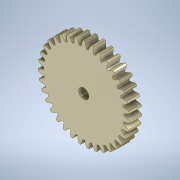
# Autodesk Inventor part: 正齒輪1
Saved by Autodesk Inventor 2020 (Build 240168000, 168)
## iProperties
CustomPartVersion: 1
Created: 2021-06-11
Part Number: 正齒輪1
Material: Steel
Document SubType Name: Modeling
Designer: user
Categories: <?xml version="1.0" encoding="UTF-16"?> <MemberInstance><Categories><FamilyTemplate><FamilyTemplateParameter ValueType="xs:double" Id="1" ObjectReferenceKey="da_z" ObjectType="kUserParameterObject"/><FamilyTemplateParameter ValueType="xs:double" Id="2" ObjectReferenceKey="da_b" ObjectType="kUserParameterObject"/><FamilyTemplateParameter ValueType="xs:double" Id="3" ObjectReferenceKey="da_beta" ObjectType="kUserParameterObject"/><FamilyTemplateParameter ValueType="xs:double" Id="4" ObjectReferenceKey="da_da" ObjectType="kUserParameterObject"/><FamilyTemplateParameter ValueType="xs:double" Id="5" ObjectReferenceKey="da_aw" ObjectType="kUserParameterObject"/><FamilyTemplateParameter ValueType="xs:string" Id="6" ObjectReferenceKey="EAIAABAAAACIAQAAAAAAAIAAAAAAAAAA" ObjectType="83910656" SubObjectId="SurfaceGeometry"/></FamilyTemplate><ParamToTemplateMap><ParamToTemplate CategoryParameter="//CategoryParameter[@InternalName='046C89C9-8512-4d59-83FE-43B91F4F132A']" TemplateParameter="1"/><ParamToTemplate CategoryParameter="//CategoryParameter[@InternalName='2552DF32-E462-4b46-AEBF-C6C7768E72AC']" TemplateParameter="2"/><ParamToTemplate CategoryParameter="//CategoryParameter[@InternalName='C9EE641D-15FC-4fae-A226-E94C4372FDD7']" TemplateParameter="3"/><ParamToTemplate><ParamToTemplate CategoryParameter="//CategoryParameter[@InternalName='00B6519A-459B-49c7-AD84-2E56D39A5744']" ConstantValue="0.000000"/></ParamToTemplate><ParamToTemplate><ParamToTemplate CategoryParameter="//CategoryParameter[@InternalName='04B31F0E-C7A6-4894-AA32-9629BEFACF47']" ConstantValue="1.000000"/></ParamToTemplate><ParamToTemplate><ParamToTemplate CategoryParameter="//CategoryParameter[@InternalName='43CBEC2E-7847-49e7-A936-2F7889FCB2D9']" ConstantValue="0.250000"/></ParamToTemplate><ParamToTemplate><ParamToTemplate CategoryParameter="//CategoryParameter[@InternalName='B1EFC894-105D-4ebd-86BF-FA20ED196853']" ConstantValue="0.350000"/></ParamToTemplate><ParamToTemplate><ParamToTemplate CategoryParameter="//CategoryParameter[@InternalName='51175063-3D10-4879-93E8-6246FE8B403D']" ConstantValue="2060000000.000000"/></ParamToTemplate><ParamToTemplate><ParamToTemplate CategoryParameter="//CategoryParameter[@InternalName='A3A52E27-4454-46a9-B0BD-C932399B70AF']" ConstantValue="0.300000"/></ParamToTemplate><ParamToTemplate><ParamToTemplate CategoryParameter="//CategoryParameter[@InternalName='91B76062-C214-41d9-B1B9-14D2AB99603D']" ConstantValue="0.200000"/></ParamToTemplate><ParamToTemplate><ParamToTemplate CategoryParameter="//CategoryParameter[@InternalName='374E806E-8B8A-4dda-A9AA-1039D6500AD2']" ConstantValue="5.000000"/></ParamToTemplate><ParamToTemplate><ParamToTemplate CategoryParameter="//CategoryParameter[@InternalName='2D373A89-B862-43d6-8D0B-0CBF12AB9F6C']" ConstantValue="0.349066"/></ParamToTemplate><ParamToTemplate CategoryParameter="//CategoryParameter[@InternalName='37777632-D6A2-4fac-9D53-DB8ACD95C989']" TemplateParameter="4"/><ParamToTemplate CategoryParameter="//CategoryParameter[@InternalName='FD1017F1-B727-4f7e-9707-0F86F1FF9423']" TemplateParameter="5"/><ParamToTemplate><ParamToTemplate CategoryParameter="//CategoryParameter[@InternalName='9E1B4470-B2D3-4ff1-B813-535BB4CDF51A']" ConstantValue="3520000.000000"/></ParamToTemplate><ParamToTemplate><ParamToTemplate CategoryParameter="//CategoryParameter[@InternalName='F8452263-BFF6-458c-9FB1-07C4B99E95CD']" ConstantValue="11400000.000000"/></ParamToTemplate><ParamToTemplate><ParamToTemplate CategoryParameter="//CategoryParameter[@InternalName='3E3BB259-FD49-497f-8171-6EBC954A3479']" ConstantValue="2.000000"/></ParamToTemplate><ParamToTemplate CategoryParameter="//CategoryParameter[@InternalName='27C3BAF2-7550-4e4b-AE2C-0DB134B7D9B7']" TemplateParameter="6"/></ParamToTemplateMap><Category DisplayName="Gear" InternalName="DC85795E-93AB-48d5-8EEE-5A27447B64BD" Mnemonic="Gear"><CategoryParameter DisplayName="z" InternalName="046C89C9-8512-4d59-83FE-43B91F4F132A" Mnemonic="z"/><CategoryParameter DisplayName="b" InternalName="2552DF32-E462-4b46-AEBF-C6C7768E72AC" Mnemonic="b"/><CategoryParameter DisplayName="||b|" InternalName="C9EE641D-15FC-4fae-A226-E94C4372FDD7" Mnemonic="beta"/><CategoryParameter DisplayName="x" InternalName="00B6519A-459B-49c7-AD84-2E56D39A5744" Mnemonic="x"/><CategoryParameter DisplayName="a*" InternalName="04B31F0E-C7A6-4894-AA32-9629BEFACF47" Mnemonic="a"/><CategoryParameter DisplayName="c*" InternalName="43CBEC2E-7847-49e7-A936-2F7889FCB2D9" Mnemonic="c"/><CategoryParameter DisplayName="r|.f|*" InternalName="B1EFC894-105D-4ebd-86BF-FA20ED196853" Mnemonic="rf"/><CategoryParameter DisplayName="E" InternalName="51175063-3D10-4879-93E8-6246FE8B403D" Mnemonic="E"/><CategoryParameter DisplayName="||m|" InternalName="A3A52E27-4454-46a9-B0BD-C932399B70AF" Mnemonic="mi"/><Category DisplayName="SpurGear" InternalName="26C5A22E-A91E-4dfd-A3B3-23CCAFAE1764" Mnemonic="SpurGear"><CategoryParameter DisplayName="m" InternalName="91B76062-C214-41d9-B1B9-14D2AB99603D" Mnemonic="m"/><CategoryParameter DisplayName="P" InternalName="374E806E-8B8A-4dda-A9AA-1039D6500AD2" Mnemonic="PP"/><CategoryParameter DisplayName="||a|" InternalName="2D373A89-B862-43d6-8D0B-0CBF12AB9F6C" Mnemonic="alpha"/><CategoryParameter DisplayName="d|.a|" InternalName="37777632-D6A2-4fac-9D53-DB8ACD95C989" Mnemonic="da"/><CategoryParameter DisplayName="a|.w|" InternalName="FD1017F1-B727-4f7e-9707-0F86F1FF9423" Mnemonic="aw"/><CategoryParameter DisplayName="||s||.Flim|" InternalName="9E1B4470-B2D3-4ff1-B813-535BB4CDF51A" Mnemonic="sFlim"/><CategoryParameter DisplayName="||s||.Hlim|" InternalName="F8452263-BFF6-458c-9FB1-07C4B99E95CD" Mnemonic="sHlim"/><CategoryParameter DisplayName="類型" InternalName="3E3BB259-FD49-497f-8171-6EBC954A3479" Mnemonic="type"/><CategoryParameter DisplayName="PitchDiameter" InternalName="27C3BAF2-7550-4e4b-AE2C-0DB134B7D9B7" Mnemonic="IDS_PITCHDIAM"/></Category></Category></Categories></MemberInstance>
Density: 1 g/cm^3
Appearance: 鎳
Author: user
Autodesk Inventor part; units mm, degrees
sketch "Sketch1" plane through (0, 0, 0) normal (0, 0, 1) x (1, 0, 0)
  circle A0 centre (0, 0) radius 37
  dimension "d0" = 74
  constraints: 1 centre point
  measures "d0" diameter of A0
extrude "Extrusion1" add sketch "Sketch1" along normal blind 20
ref_plane "Work Plane2" through (0, 0, 10) normal (0, 0, 1) x (1, 0, 0)
sketch "Sketch2" plane through (0, 0, 0) normal (0, 0, -1) x (-1, 0, 0)
  circle A0 centre (0, 0) radius 37 projected
  circle A1 centre (0, 0) radius 35
  dimension "d3" = 70
  constraints: 1 centre point, 1 coincident
  measures "d3" diameter of A1
surface extrude "節圓直徑" sketch "Sketch2" against normal through all shown no curves A1
ref_plane "Work Plane8" through (0, 0, 0) normal (0.9959743, 0.0896393, 0) x (0, 0, 1)
ref_plane "Work Plane9" through (0, 0, 0) normal (1, 0, 0) x (0, 1, 0)
spur gear teeth "正齒輪" teeth 35 pitch diameter 70 tip diameter 74 root diameter 65 face width 20 start plane through (0, 0, 0) normal (0, 0, -1) x (-1, 0, 0)
sketch "草圖3" plane through (0, 0, 20) normal (0, 0, 1) x (1, 0, 0)
  line L0 (-1.995, -3.467) -> (1.688, -3.6264) projected
  arc A0 (1.688, -3.6264) -> (-1.995, -3.467) centre (0, 0) ccw projected
  point P0 (0, 0)
ref_plane "工作平面11" through (-40.6499, -40.6499, -1.2) normal (0, 0, -1) x (0.0432397, 0.9990647, 0)
extrude "擠出2" cut sketch "草圖3" against normal up to surface (21.2 mm away)
sketch "草圖4" plane through (0, 0, 20) normal (0, 0, 1) x (1, 0, 0)
  line L0 (1.688, -3.6264) -> (-1.995, -3.467) projected
  arc A0 (1.688, -3.6264) -> (-1.995, -3.467) centre (0, 0) ccw projected
  arc A1 (-7.4218, 36.248) -> (-7.9411, 31.5149) centre (13.3274, 31.5766) ccw projected
  arc A2 (-7.9411, 31.5149) -> (-9.347, 31.1269) centre (0, 0) ccw projected
  arc A3 (-9.347, 31.1269) -> (-12.2203, 34.9237) centre (-27.6365, 20.2713) ccw projected
  arc A4 (-12.2203, 34.9237) -> (-13.7749, 34.3403) centre (0, 0) ccw projected
  arc A5 (-13.7749, 34.3403) -> (-13.4407, 29.5905) centre (7.475, 33.4489) ccw projected
  arc A6 (-13.4407, 29.5905) -> (-14.7547, 28.9577) centre (0, 0) ccw projected
  arc A7 (-14.7547, 28.9577) -> (-18.2598, 32.1804) centre (-30.812, 15.0108) ccw projected
  arc A8 (-18.2598, 32.1804) -> (-19.6852, 31.3288) centre (0, 0) ccw projected
  arc A9 (-19.6852, 31.3288) -> (-18.5082, 26.7151) centre (1.3824, 34.2461) ccw projected
  arc A10 (-18.5082, 26.7151) -> (-19.6882, 25.8578) centre (0, 0) ccw projected
  arc A11 (-19.6882, 25.8578) -> (-23.7124, 28.4029) centre (-32.9971, 9.2679) ccw projected
  arc A12 (-23.7124, 28.4029) -> (-24.9628, 27.3104) centre (0, 0) ccw projected
  arc A13 (-24.9628, 27.3104) -> (-22.981, 22.981) centre (-4.7547, 33.9425) ccw projected
  arc A14 (-22.981, 22.981) -> (-23.9889, 21.9268) centre (0, 0) ccw projected
  arc A15 (-23.9889, 21.9268) -> (-28.4029, 23.7124) centre (-34.1217, 3.2271) ccw projected
  arc A16 (-28.4029, 23.7124) -> (-29.4381, 22.4142) centre (0, 0) ccw projected
  arc A17 (-29.4381, 22.4142) -> (-26.7151, 18.5082) centre (-10.739, 32.5481) ccw projected
  arc A18 (-26.7151, 18.5082) -> (-27.5185, 17.291) centre (0, 0) ccw projected
  arc A19 (-27.5185, 17.291) -> (-32.1804, 18.2598) centre (-34.1496, -2.9174) ccw projected
  arc A20 (-32.1804, 18.2598) -> (-32.9672, 16.7976) centre (0, 0) ccw projected
  arc A21 (-32.9672, 16.7976) -> (-29.5905, 13.4407) centre (-16.3781, 30.1075) ccw projected
  arc A22 (-29.5905, 13.4407) -> (-30.1637, 12.0995) centre (0, 0) ccw projected
  arc A23 (-30.1637, 12.0995) -> (-34.9237, 12.2203) centre (-33.0798, -8.9682) ccw projected
  arc A24 (-34.9237, 12.2203) -> (-35.4368, 10.6412) centre (0, 0) ccw projected
  arc A25 (-35.4368, 10.6412) -> (-31.5149, 7.9411) centre (-21.4908, 26.6992) ccw projected
  arc A26 (-31.5149, 7.9411) -> (-31.8395, 6.5192) centre (0, 0) ccw projected
  arc A27 (-31.8395, 6.5192) -> (-36.5445, 5.7881) centre (-30.9469, -14.7307) ccw projected
  arc A28 (-36.5445, 5.7881) -> (-36.7674, 4.1427) centre (0, 0) ccw projected
  arc A29 (-36.7674, 4.1427) -> (-32.4264, 2.1862) centre (-25.9127, 22.4329) ccw projected
  arc A30 (-32.4264, 2.1862) -> (-32.4918, 0.7292) centre (0, 0) ccw projected
  arc A31 (-32.4918, 0.7292) -> (-36.9907, -0.8302) centre (-27.8193, -20.0197) ccw projected
  arc A32 (-36.9907, -0.8302) -> (-36.9162, -2.489) centre (0, 0) ccw projected
  arc A33 (-36.9162, -2.489) -> (-32.2956, -3.6388) centre (-29.5019, 17.4454) ccw projected
  arc A34 (-32.2956, -3.6388) -> (-32.0999, -5.0841) centre (0, 0) ccw projected
  arc A35 (-32.0999, -5.0841) -> (-36.248, -7.4218) centre (-23.7976, -24.6653) ccw projected
  arc A36 (-36.248, -7.4218) -> (-35.8785, -9.0406) centre (0, 0) ccw projected
  arc A37 (-35.8785, -9.0406) -> (-31.1269, -9.347) centre (-32.1428, 11.8973) ccw projected
  arc A38 (-31.1269, -9.347) -> (-30.6762, -10.7341) centre (0, 0) ccw projected
  arc A39 (-30.6762, -10.7341) -> (-34.3403, -13.7749) centre (-19.011, -28.5182) ccw projected
  arc A40 (-34.3403, -13.7749) -> (-33.6877, -15.3017) centre (0, 0) ccw projected
  arc A41 (-33.6877, -15.3017) -> (-28.9577, -14.7547) centre (-33.7506, 5.9668) ccw projected
  arc A42 (-28.9577, -14.7547) -> (-28.2666, -16.039) centre (0, 0) ccw projected
  arc A43 (-28.2666, -16.039) -> (-31.3288, -19.6852) centre (-13.6133, -31.4544) ccw projected
  arc A44 (-31.3288, -19.6852) -> (-30.4141, -21.0709) centre (0, 0) ccw projected
  arc A45 (-30.4141, -21.0709) -> (-25.8578, -19.6882) centre (-34.2736, -0.1555) ccw projected
  arc A46 (-25.8578, -19.6882) -> (-24.9485, -20.8285) centre (0, 0) ccw projected
  arc A47 (-24.9485, -20.8285) -> (-27.3104, -24.9628) centre (-7.7782, -33.3797) ccw projected
  arc A48 (-27.3104, -24.9628) -> (-26.163, -26.163) centre (0, 0) ccw projected
  arc A49 (-26.163, -26.163) -> (-21.9268, -23.9889) centre (-33.695, -6.2727) ccw projected
  arc A50 (-21.9268, -23.9889) -> (-20.8285, -24.9485) centre (0, 0) ccw projected
  arc A51 (-20.8285, -24.9485) -> (-22.4142, -29.4381) centre (-1.693, -34.2321) ccw projected
  arc A52 (-22.4142, -29.4381) -> (-21.0709, -30.4141) centre (0, 0) ccw projected
  arc A53 (-21.0709, -30.4141) -> (-17.291, -27.5185) centre (-32.0335, -12.1884) ccw projected
  arc A54 (-17.291, -27.5185) -> (-16.039, -28.2666) centre (0, 0) ccw projected
  arc A55 (-16.039, -28.2666) -> (-16.7976, -32.9672) centre (4.4466, -33.9843) ccw projected
  arc A56 (-16.7976, -32.9672) -> (-15.3017, -33.6877) centre (0, 0) ccw projected
  arc A57 (-15.3017, -33.6877) -> (-12.0995, -30.1637) centre (-29.3424, -17.7124) ccw projected
  arc A58 (-12.0995, -30.1637) -> (-10.7341, -30.6762) centre (0, 0) ccw projected
  arc A59 (-10.7341, -30.6762) -> (-10.6412, -35.4368) centre (10.4433, -32.6442) ccw projected
  arc A60 (-10.6412, -35.4368) -> (-9.0406, -35.8785) centre (0, 0) ccw projected
  arc A61 (-9.0406, -35.8785) -> (-6.5192, -31.8395) centre (-25.7082, -22.667) ccw projected
  arc A62 (-6.5192, -31.8395) -> (-5.0841, -32.0999) centre (0, 0) ccw projected
  arc A63 (-5.0841, -32.0999) -> (-4.1427, -36.7674) centre (16.1043, -30.2548) ccw projected
  arc A64 (-4.1427, -36.7674) -> (-2.489, -36.9162) centre (0, 0) ccw projected
  arc A65 (-2.489, -36.9162) -> (-0.7292, -32.4918) centre (-21.2477, -26.8931) ccw projected
  arc A66 (-0.7292, -32.4918) -> (0.7292, -32.4918) centre (0, 0) ccw projected
  arc A67 (0.7292, -32.4918) -> (2.489, -36.9162) centre (21.2477, -26.8931) ccw projected
  arc A68 (2.489, -36.9162) -> (4.1427, -36.7674) centre (0, 0) ccw projected
  arc A69 (4.1427, -36.7674) -> (5.0841, -32.0999) centre (-16.1043, -30.2548) ccw projected
  arc A70 (5.0841, -32.0999) -> (6.5192, -31.8395) centre (0, 0) ccw projected
  arc A71 (6.5192, -31.8395) -> (9.0406, -35.8785) centre (25.7082, -22.667) ccw projected
  arc A72 (9.0406, -35.8785) -> (10.6412, -35.4368) centre (0, 0) ccw projected
  arc A73 (10.6412, -35.4368) -> (10.7341, -30.6762) centre (-10.4433, -32.6442) ccw projected
  arc A74 (10.7341, -30.6762) -> (12.0995, -30.1637) centre (0, 0) ccw projected
  arc A75 (12.0995, -30.1637) -> (15.3017, -33.6877) centre (29.3424, -17.7124) ccw projected
  arc A76 (15.3017, -33.6877) -> (16.7976, -32.9672) centre (0, 0) ccw projected
  arc A77 (16.7976, -32.9672) -> (16.039, -28.2666) centre (-4.4466, -33.9843) ccw projected
  arc A78 (16.039, -28.2666) -> (17.291, -27.5185) centre (0, 0) ccw projected
  arc A79 (17.291, -27.5185) -> (21.0709, -30.4141) centre (32.0335, -12.1884) ccw projected
  arc A80 (21.0709, -30.4141) -> (22.4142, -29.4381) centre (0, 0) ccw projected
  arc A81 (22.4142, -29.4381) -> (20.8285, -24.9485) centre (1.693, -34.2321) ccw projected
  arc A82 (20.8285, -24.9485) -> (21.9268, -23.9889) centre (0, 0) ccw projected
  arc A83 (21.9268, -23.9889) -> (26.163, -26.163) centre (33.695, -6.2727) ccw projected
  arc A84 (26.163, -26.163) -> (27.3104, -24.9628) centre (0, 0) ccw projected
  arc A85 (27.3104, -24.9628) -> (24.9485, -20.8285) centre (7.7782, -33.3797) ccw projected
  arc A86 (24.9485, -20.8285) -> (25.8578, -19.6882) centre (0, 0) ccw projected
  arc A87 (25.8578, -19.6882) -> (30.4141, -21.0709) centre (34.2736, -0.1555) ccw projected
  arc A88 (30.4141, -21.0709) -> (31.3288, -19.6852) centre (0, 0) ccw projected
  arc A89 (31.3288, -19.6852) -> (28.2666, -16.039) centre (13.6133, -31.4544) ccw projected
  arc A90 (28.2666, -16.039) -> (28.9577, -14.7547) centre (0, 0) ccw projected
  arc A91 (28.9577, -14.7547) -> (33.6877, -15.3017) centre (33.7506, 5.9668) ccw projected
  arc A92 (33.6877, -15.3017) -> (34.3403, -13.7749) centre (0, 0) ccw projected
  arc A93 (34.3403, -13.7749) -> (30.6762, -10.7341) centre (19.011, -28.5182) ccw projected
  arc A94 (30.6762, -10.7341) -> (31.1269, -9.347) centre (0, 0) ccw projected
  arc A95 (31.1269, -9.347) -> (35.8785, -9.0406) centre (32.1428, 11.8973) ccw projected
  arc A96 (35.8785, -9.0406) -> (36.248, -7.4218) centre (0, 0) ccw projected
  arc A97 (36.248, -7.4218) -> (32.0999, -5.0841) centre (23.7976, -24.6653) ccw projected
  arc A98 (32.0999, -5.0841) -> (32.2956, -3.6388) centre (0, 0) ccw projected
  arc A99 (32.2956, -3.6388) -> (36.9162, -2.489) centre (29.5019, 17.4454) ccw projected
  arc A100 (36.9162, -2.489) -> (36.9907, -0.8302) centre (0, 0) ccw projected
  arc A101 (36.9907, -0.8302) -> (32.4918, 0.7292) centre (27.8193, -20.0197) ccw projected
  arc A102 (32.4918, 0.7292) -> (32.4264, 2.1862) centre (0, 0) ccw projected
  arc A103 (32.4264, 2.1862) -> (36.7674, 4.1427) centre (25.9127, 22.4329) ccw projected
  arc A104 (36.7674, 4.1427) -> (36.5445, 5.7881) centre (0, 0) ccw projected
  arc A105 (36.5445, 5.7881) -> (31.8395, 6.5192) centre (30.9469, -14.7307) ccw projected
  arc A106 (31.8395, 6.5192) -> (31.5149, 7.9411) centre (0, 0) ccw projected
  arc A107 (31.5149, 7.9411) -> (35.4368, 10.6412) centre (21.4908, 26.6992) ccw projected
  arc A108 (35.4368, 10.6412) -> (34.9237, 12.2203) centre (0, 0) ccw projected
  arc A109 (34.9237, 12.2203) -> (30.1637, 12.0995) centre (33.0798, -8.9682) ccw projected
  arc A110 (30.1637, 12.0995) -> (29.5905, 13.4407) centre (0, 0) ccw projected
  arc A111 (29.5905, 13.4407) -> (32.9672, 16.7976) centre (16.3781, 30.1075) ccw projected
  arc A112 (32.9672, 16.7976) -> (32.1804, 18.2598) centre (0, 0) ccw projected
  arc A113 (32.1804, 18.2598) -> (27.5185, 17.291) centre (34.1496, -2.9174) ccw projected
  arc A114 (27.5185, 17.291) -> (26.7151, 18.5082) centre (0, 0) ccw projected
  arc A115 (26.7151, 18.5082) -> (29.4381, 22.4142) centre (10.739, 32.5481) ccw projected
  arc A116 (29.4381, 22.4142) -> (28.4029, 23.7124) centre (0, 0) ccw projected
  arc A117 (28.4029, 23.7124) -> (23.9889, 21.9268) centre (34.1217, 3.2271) ccw projected
  arc A118 (23.9889, 21.9268) -> (22.981, 22.981) centre (0, 0) ccw projected
  arc A119 (22.981, 22.981) -> (24.9628, 27.3104) centre (4.7547, 33.9425) ccw projected
  arc A120 (24.9628, 27.3104) -> (23.7124, 28.4029) centre (0, 0) ccw projected
  arc A121 (23.7124, 28.4029) -> (19.6882, 25.8578) centre (32.9971, 9.2679) ccw projected
  arc A122 (19.6882, 25.8578) -> (18.5082, 26.7151) centre (0, 0) ccw projected
  arc A123 (18.5082, 26.7151) -> (19.6852, 31.3288) centre (-1.3824, 34.2461) ccw projected
  arc A124 (19.6852, 31.3288) -> (18.2598, 32.1804) centre (0, 0) ccw projected
  arc A125 (18.2598, 32.1804) -> (14.7547, 28.9577) centre (30.812, 15.0108) ccw projected
  arc A126 (14.7547, 28.9577) -> (13.4407, 29.5905) centre (0, 0) ccw projected
  arc A127 (13.4407, 29.5905) -> (13.7749, 34.3403) centre (-7.475, 33.4489) ccw projected
  arc A128 (13.7749, 34.3403) -> (12.2203, 34.9237) centre (0, 0) ccw projected
  arc A129 (12.2203, 34.9237) -> (9.347, 31.1269) centre (27.6365, 20.2713) ccw projected
  arc A130 (9.347, 31.1269) -> (7.9411, 31.5149) centre (0, 0) ccw projected
  arc A131 (7.9411, 31.5149) -> (7.4218, 36.248) centre (-13.3274, 31.5766) ccw projected
  arc A132 (7.4218, 36.248) -> (5.7881, 36.5445) centre (0, 0) ccw projected
  arc A133 (5.7881, 36.5445) -> (3.6388, 32.2956) centre (23.5728, 24.8802) ccw projected
  arc A134 (3.6388, 32.2956) -> (2.1862, 32.4264) centre (0, 0) ccw projected
  arc A135 (2.1862, 32.4264) -> (0.8302, 36.9907) centre (-18.7515, 28.6895) ccw projected
  arc A136 (0.8302, 36.9907) -> (-0.8302, 36.9907) centre (0, 0) ccw projected
  arc A137 (-0.8302, 36.9907) -> (-2.1862, 32.4264) centre (18.7515, 28.6895) ccw projected
  arc A138 (-2.1862, 32.4264) -> (-3.6388, 32.2956) centre (0, 0) ccw projected
  arc A139 (-3.6388, 32.2956) -> (-5.7881, 36.5445) centre (-23.5728, 24.8802) ccw projected
  arc A140 (-5.7881, 36.5445) -> (-7.4218, 36.248) centre (0, 0) ccw projected
extrude "擠出3" cut sketch "草圖4" against normal blind 10
equation "\"d0\" = da_da"
equation "\"d1\" = da_b"
equation "\"d3\" = da_dw"
equation "\"da_da\" = 74"
equation "\"da_b\" = 20"
equation "\"da_dw\" = 70"
body "Solid1"
body "Srf1"
